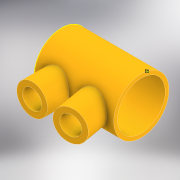
# Autodesk Inventor part: SoporteMotor
Saved by Autodesk Inventor 2021 (Build 250183000, 183)
## iProperties
Created: 2024-02-19
Part Number: SoporteMotor
Material: PLA
Document SubType Name: Modeling
Designer: Martin
Density: 1.27 g/cm^3
Appearance: PLA
Mass: 54.1176 g
Surface Area: 250.747 cm^2
Volume: 42.6123 cm^3
Author: Martin
Autodesk Inventor part; units mm, degrees
ref_plane "YZ Plane" through (0, 0, 0) normal (1, 0, 0) x (0, 1, 0)
ref_plane "XZ Plane" through (0, 0, 0) normal (0, 1, 0) x (-1, 0, 0)
ref_plane "XY Plane" through (0, 0, 0) normal (0, 0, 1) x (1, 0, 0)
sketch "Sketch2" plane through (0, 0, 0) normal (1, 0, 0) x (0, 1, 0)
  circle A0 centre (0, 0) radius 19.5
  circle A1 centre (0, 0) radius 22.5
  dimension "d0" = 39
  dimension "d1" = 45
  constraints: 2 centre point, 2 coincident
  measures "d0" diameter of A0
  measures "d1" diameter of A1
extrude "Extrusion1" add sketch "Sketch2" along normal mid plane 65 contours A0 | A1
sketch "Sketch3" plane through (32.5, 0, 0) normal (1, 0, 0) x (0, 0, -1)
  circle A0 centre (0, 0) radius 19.5
  dimension "d4" = 39
  constraints: 1 centre point, 1 coincident
  measures "d4" diameter of A0
extrude "Extrusion2" cut sketch "Sketch3" against normal blind 60
sketch "Sketch4" plane through (-32.5, 0, 0) normal (-1, 0, 0) x (0, 0, 1)
  circle A0 centre (-15.7, 0) radius 2
  point P0 (0, 0)
  point P1 (0, 0)
  dimension "d7" = 4
  dimension "d45" = 15.7
  constraints: 2 coincident, 1 centre point
  measures "d7" diameter of A0
  measures "d45" distance of point (0, 0) A0.centre
extrude "Extrusion3" cut sketch "Sketch4" against normal blind 5
pattern_circular "Circular Pattern1" count 6 over 360 about axis through (-10, 0, 0) along (1, 0, 0) of "Extrusion3"
sketch "Sketch5" plane through (-32.5, 0, 0) normal (-1, 0, 0) x (0, 0, 1)
  circle A0 centre (0, -7.11) radius 6.5
  point P0 (0, 0)
  dimension "d13" = 13
  constraints: 1 centre point, 1 coincident
  measures "d13" diameter of A0
extrude "Extrusion4" cut sketch "Sketch5" against normal blind 5
ref_plane "Work Plane1" through (0, 0, 40) normal (0, 0, 1) x (1, 0, 0)
sketch "Sketch6" plane through (0, 0, 40) normal (0, 0, 1) x (1, 0, 0)
  circle A0 centre (-16.4979, 0) radius 12.5
  circle A1 centre (-16.4979, 0) radius 7.9
  point P0 (0, 0)
  dimension "d17" = 25
  dimension "d18" = 15.8
  constraints: 2 centre point, 1 coincident
  measures "d17" diameter of A0
  measures "d18" diameter of A1
extrude "Extrusion5" add sketch "Sketch6" against normal up to surface round surface about axis through (0, 0, 0) along (1, 0, 0) radius 22.5 far side no
sketch "Sketch7" plane through (0, 0, 40) normal (0, 0, 1) x (1, 0, 0)
  line L0 (32.5, -22.5) -> (32.5, 22.5) projected
  point P0 (0, 0)
ref_plane "Work Plane2" through (32.5, -22.5, 40) normal (0.1736482, 0, 0.9848078) x (0, 1, 0)
sketch "Sketch8" plane through (32.5, -22.5, 40) normal (0.1736482, 0, 0.9848078) x (0, 1, 0)
  circle A0 centre (22.5, 15.2535) radius 12.5
  circle A1 centre (22.5, 15.2535) radius 7.9
  ellipse E0 centre (22.5, 48.2535) end of major axis (30.4, 48.2535) minor radius 7.78 projected
  point P0 (22.5, 25.0603)
  dimension "d22" = 25
  dimension "d23" = 15.8
  dimension "d26" = 33
  constraints: 2 centre point, 1 coincident
  measures "d22" diameter of A0
  measures "d23" diameter of A1
  measures "d26" distance of A0.centre E0.centre
extrude "Extrusion6" add sketch "Sketch8" against normal up to surface contours A0 round surface about axis through (0, 0, 0) along (1, 0, 0) radius 22.5 far side no
sketch "Sketch9" plane through (-32.5, 0, 0) normal (-1, 0, 0) x (0, 0, 1)
  circle A0 centre (0, -7.11) radius 6.5 projected
  circle A1 centre (-7.85, -13.5966) radius 2 projected
  circle A2 centre (7.85, -13.5966) radius 2 projected
  circle A3 centre (15.7, 0) radius 2 projected
  circle A4 centre (7.85, 13.5966) radius 2 projected
  circle A5 centre (-7.85, 13.5966) radius 2 projected
  circle A6 centre (-15.7, 0) radius 2 projected
  circle A7 centre (0, 0) radius 22.5 projected
body "Solid1"
